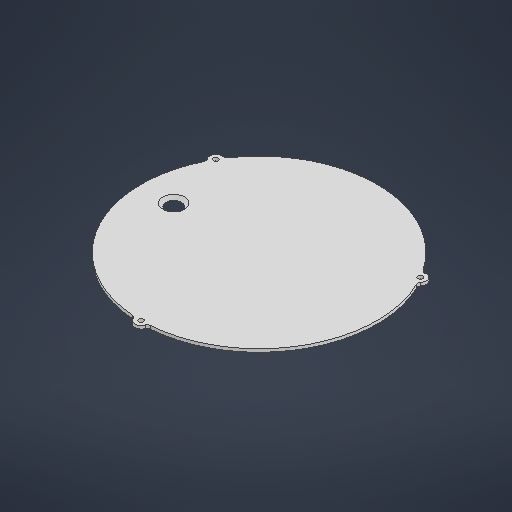
# Autodesk Inventor part: Vial Cover
Saved by Autodesk Inventor 2025.1 (Build 291241000, 241)
## iProperties
Created: 2025-02-24
Part Number: Vial Cover
Material: Generic
Document SubType Name: Modeling
Designer: jerem
Density: 1 g/cm^3
Appearance: Default
Author: jerem
## iProperties of the stored document Vial Cover_3DPrint.ipt
Created: 2025-02-24
Part Number: Vial Cover_3DPrint
Material: Generic
Document SubType Name: Modeling
Designer: jerem
Density: 1 g/cm^3
Appearance: Default
Author: jerem
Autodesk Inventor part; units mm, degrees
ref_plane "YZ Plane" through (0, 0, 0) normal (1, 0, 0) x (0, 1, 0)
ref_plane "XZ Plane" through (0, 0, 0) normal (0, 1, 0) x (-1, 0, 0)
ref_plane "XY Plane" through (0, 0, 0) normal (0, 0, 1) x (1, 0, 0)
sketch "Sketch1" plane through (0, 0, 0) normal (0, 1, 0) x (-1, 0, 0)
  circle A0 centre (0, 0) radius 70
  circle A1 centre (55, 0) radius 5
  line L0 (55, 0) -> (0, 0) construction
  line L1 (0, 0) -> (0, 70) construction
  circle A2 centre (0, 76) radius 1.6
  line L2 (0, 76) -> (0, 70) construction
  circle A3 centre (0, 0) radius 76
  circle A4 centre (0, 76) radius 4
  circle A5 centre (65.8179, -38) radius 4
  circle A6 centre (65.8179, -38) radius 1.6
  circle A7 centre (-65.8179, -38) radius 4
  circle A8 centre (-65.8179, -38) radius 1.6
  point P0 (-1.5999, 75.9832)
  point P1 (1.5999, 75.9832)
  point P2 (3.9986, 75.8947)
  point P3 (-3.9986, 75.8947)
  point P4 (63.7275, -41.4103)
  point P5 (67.7261, -34.4845)
  point P6 (-67.7261, -34.4845)
  point P7 (-63.7275, -41.4103)
  dimension "d0" = 140
  dimension "d1" = 10
  dimension "d2" = 55
  dimension "d9" = 3.2
  dimension "d25" = 6
  dimension "d26" = 76
  dimension "d27" = 8
  dimension "d33" = 360
  constraints: 8 centre point, 6 end point, 4 coincident, 2 vertical, 1 horizontal, 1 vertical alignment, 15 other
  measures "d1" diameter of A1
  measures "d2" distance of L0.start L0.end
  measures "d9" diameter of A2
  measures "d26" distance of point (0, 0) L2.start
  measures "d27" diameter of A4
extrude "Extrusion1" add sketch "Sketch1" along normal blind 2 contours A0 | A2 A3 A4 | A2 A3 A4 | A4 A3 A5 A7 | A7 A3 A8 | A3 A8 A7 | A5 A3 A6 | A3 A6 A5
chamfer "Chamfer1" distance 2 angle 45 1 edges at (-50, 2, 0)
fillet "Fillet1" radius 2 6 edges at (-3.9986, 1, 75.8947) (3.9986, 1, 75.8947) (67.7261, 1, -34.4845) (63.7275, 1, -41.4103) (-63.7275, 1, -41.4103) (-67.7261, 1, -34.4845)
body "Solid1"
